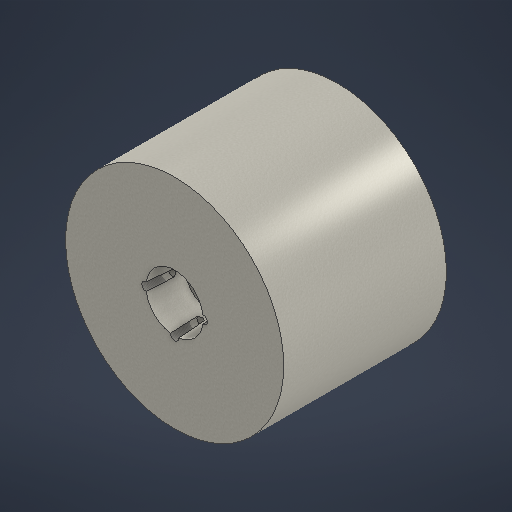
# Autodesk Inventor part: Masse
Saved by Autodesk Inventor 2026.2 (Build 302298010, 298A)
## iProperties
Created: 2026-04-11
Part Number: Masse
Material: Générique
Document SubType Name: Modeling
Designer: romai
Density: 1 g/cm^3
Appearance: Par défaut
Author: romai
Autodesk Inventor part; units mm, degrees
ref_plane "YZ Plane" through (0, 0, 0) normal (1, 0, 0) x (0, 1, 0)
ref_plane "XZ Plane" through (0, 0, 0) normal (0, 1, 0) x (-1, 0, 0)
ref_plane "XY Plane" through (0, 0, 0) normal (0, 0, 1) x (1, 0, 0)
sketch "Esquisse3" plane through (0, 0, 0) normal (1, 0, 0) x (0, 1, 0)
  line L0 (12.5, 50) -> (17.6, 50)
  line L1 (12.5, 27.7) -> (16, 27.7)
  line L2 (16, 27.7) -> (17.6, 50)
  line L3 (-39.3437, 0) -> (46.6159, 0)
  line L4 (12.5, -50) -> (17.6, -50)
  line L5 (12.5, -27.7) -> (16, -27.7)
  line L6 (16, -27.7) -> (17.6, -50)
  line L7 (12.5, -50) -> (12.5, -27.7)
  line L8 (0, 98.6871) -> (0, -122.4022)
  line L9 (17.6, 50) -> (67, 50)
  line L10 (67, 50) -> (67, -50)
  line L11 (67, -50) -> (17.6, -50)
  line L12 (12.5, 50) -> (12.5, 27.7)
  line L13 (12.5, 27.7) -> (12.5, -27.7)
  point P0 (0, 0)
  point P1 (40.7356, 59.8426)
  point P2 (56.7464, 59.8426)
  point P3 (58.3249, 81.8426)
  point P4 (40.7356, 81.8426)
  dimension "d14" = 22.3
  dimension "d19" = 0
  dimension "d20" = 100
  dimension "d21" = 0
  dimension "d22" = 25
  dimension "d23" = 134
  dimension "d25" = 35.2
  dimension "d26" = 32
  constraints: 28 end point, 4 horizontal, 4 symmetric about line, 3 vertical, 2 perpendicular, 1 collinear
  measures "d14" distance between parallel lines of L1 L0
  measures "d19" distance from line of point (0, 0) L8
  measures "d20" distance of L6.end L0.end
  measures "d21" distance from line of point (0, 0) L3
  measures "d22" diameter of L12 L8
  measures "d23" diameter of L10 L8
  measures "d25" diameter of L0.end L8
  measures "d26" diameter of L1.end L8
revolve "Révolution1" add sketch "Esquisse3" angle 360 about axis through (0, 0, 98.6871) along (0, 0, -1) contours L9 L10 L11 L6 L5 L13 L1 L2
sketch "Esquisse4" plane through (0, 0, 50) normal (0, 0, 1) x (1, 0, 0)
  circle A0 centre (0, 0) radius 17.6 projected
  line L0 (-27.4685, -0.0852) -> (22.7682, -0.0852)
  line L1 (0, 22.4796) -> (0, -21.2618)
  point P0 (0, 0)
  point P1 (17.5998, -0.0852)
  point P2 (0, -17.6)
  point P3 (-17.5998, -0.0852)
  constraints: 4 end point, 3 point on circle, 3 point on line, 1 horizontal, 1 vertical
hole "Perçage2" at (17.5998, -0.0852, 50) at (0, -17.6, 50) at (-17.5998, -0.0852, 50) direction (0, 0, -1) diameter 5.134 depth 16.2 tip angle 118 thread size "M6x0.8" class "6H" standard "ISO Metric profile"
mirror "Mise en miroir1" about plane through (0, 0, 0) normal (0, 0, 1) of "Perçage2"
